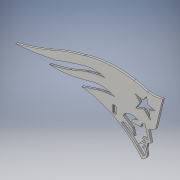
# Autodesk Inventor part: RTS patriots
Saved by Autodesk Inventor 2016 (Build 200138000, 138)
## iProperties
Created: 2017-12-19
Part Number: RTS patriots
Material: Generic
Document SubType Name: Modeling
Designer: student
Density: 1 g/cm^3
Appearance: Default
Author: student
Autodesk Inventor part; units mm, degrees
ref_plane "YZ Plane" through (0, 0, 0) normal (1, 0, 0) x (0, 1, 0)
ref_plane "XZ Plane" through (0, 0, 0) normal (0, 1, 0) x (-1, 0, 0)
ref_plane "XY Plane" through (0, 0, 0) normal (0, 0, 1) x (1, 0, 0)
sketch "Sketch1" plane through (0, 0, 0) normal (0, 0, 1) x (1, 0, 0)
  line L0 (-121.92, 53.34) -> (121.92, 53.34)
  line L1 (121.92, 53.34) -> (121.92, -53.34)
  line L2 (121.92, -53.34) -> (-121.92, -53.34)
  line L3 (-121.92, -53.34) -> (-121.92, 53.34)
  line L4 (-121.92, 53.34) -> (121.92, -53.34) construction
  line L5 (121.92, 53.34) -> (-121.92, -53.34) construction
  arc A0 (67.5496, -52.2242) -> (-16.5252, -5.911) centre (-36.2594, -141.2049) ccw
  arc A1 (67.5496, -52.2242) -> (78.4495, -31.764) centre (64.7451, -37.5966) ccw
  arc A2 (-20.2647, 1.2126) -> (-16.5252, -5.911) centre (-17.1494, -1.6953) ccw
  arc A3 (-43.7287, -2.3938) -> (-20.2647, 1.2126) centre (-53.1153, 136.8126) ccw
  arc A4 (-61.5471, -2.0063) -> (-43.7287, -2.3938) centre (-51.0941, 68.8006) ccw
  arc A5 (-65.9278, 3.1159) -> (-61.5471, -2.0063) centre (-61.6241, 2.3622) ccw
  arc A6 (-108.1597, -0.5066) -> (-65.9278, 3.1159) centre (-96.2599, 108.7489) ccw
  arc A7 (-109.606, 7.2871) -> (-108.1597, -0.5066) centre (-107.7116, 3.6077) ccw
  arc A8 (-109.606, 7.2871) -> (-29.7712, 36.4682) centre (-485.0256, 1158.173) ccw
  arc A9 (46.8022, 47.5707) -> (-29.7712, 36.4682) centre (33.6127, -131.0759) ccw
  arc A10 (75.8647, 41.5807) -> (46.8022, 47.5707) centre (24.6007, -133.6461) ccw
  arc A11 (75.8647, 41.5807) -> (97.0333, 43.8681) centre (82.7984, 76.5092) ccw
  arc A12 (101.3733, 39.6116) -> (97.0333, 43.8681) centre (98.7975, 41.3261) ccw
  line L6 (101.3733, 39.6116) -> (91.2149, -4.1951)
  line L7 (91.2149, -4.1951) -> (82.1219, -9.828)
  line L8 (82.1219, -9.828) -> (85.6883, -23.6524)
  line L9 (85.6883, -23.6524) -> (79.8094, -27.2942)
  line L10 (79.8094, -27.2942) -> (78.4495, -31.764)
  arc A13 (-8.123, 25.7478) -> (-50.7898, 11.8734) centre (130.1222, -471.929) ccw
  arc A14 (-59.7387, 2.1709) -> (-25.343, 4.6976) centre (-51.96, 131.6592) ccw
  arc A15 (-25.343, 4.6976) -> (-3.3955, 10.2777) centre (-241.5674, 901.0891) ccw
  arc A16 (-59.7387, 2.1709) -> (-30.5588, 10.2777) centre (-108.6142, 234.6643) ccw
  arc A17 (-6.8927, 19.9675) -> (-30.5588, 10.2777) centre (128.911, -345.4626) ccw
  arc A18 (29.71, 8.6625) -> (7.2861, 5.2273) centre (28.2796, -56.9055) ccw
  arc A19 (67.5496, -46.6147) -> (-15.043, -2.1204) centre (-26.7986, -122.8453) ccw
  arc A20 (7.2861, 5.2273) -> (-15.043, -2.1204) centre (125.1778, -390.6373) ccw
  arc A21 (29.71, 8.6625) -> (-1.7387, 10.7223) centre (11.2905, -31.4567) ccw
  arc A22 (16.6394, 24.5902) -> (-4.4734, 20.4951) centre (20.0682, -49.5605) ccw
  arc A23 (16.6394, 24.5902) -> (-6.1428, 26.0437) centre (2.4584, -18.4113) ccw
  line L11 (-4.4734, 20.4951) -> (-6.8927, 19.9675)
  line L12 (-1.7387, 10.7223) -> (-3.3955, 10.2777)
  line L13 (-8.123, 25.7478) -> (-6.1428, 26.0437)
  line L14 (-11.9813, 36.4379) -> (-9.4594, 37.5475)
  arc A24 (56.7247, 41.3261) -> (-9.4594, 37.5475) centre (32.0703, -108.3526) ccw
  arc A25 (75.5018, 36.9927) -> (96.2941, 38.7613) centre (82.101, 82.5143) ccw
  arc A26 (75.5018, 36.9927) -> (56.7247, 41.3261) centre (-574.7188, -2737.6346) ccw
  arc A27 (48.5931, -2.1204) -> (42.2239, -8.0879) centre (49.4213, -9.3871) ccw
  arc A28 (62.5792, -3.2945) -> (48.5931, -2.1204) centre (54.4536, -16.199) ccw
  arc A29 (62.5792, -3.2945) -> (53.1895, -9.828) centre (61.8675, -12.2858) ccw
  arc A30 (72.3073, -2.9923) -> (66.2757, -9.3006) centre (72.5246, -9.2377) ccw
  arc A31 (45.1126, -15.108) -> (39.2947, -17.8603) centre (44.2132, -20.7321) ccw
  arc A32 (52.8788, -19.3209) -> (45.1126, -15.108) centre (42.182, -29.7749) ccw
  arc A33 (57.5173, -24.7402) -> (52.8788, -19.3209) centre (-276.2295, -305.7101) ccw
  arc A34 (69.3744, -42.5298) -> (72.1611, -35.7997) centre (66.7227, -37.4899) ccw
  arc A35 (67.5496, -46.6147) -> (73.5131, -32.8714) centre (66.056, -37.8011) ccw
  arc A36 (72.1611, -35.7997) -> (68.1792, -31.764) centre (38.6776, -64.8546) ccw
  arc A37 (69.3744, -42.5298) -> (39.2947, -17.8603) centre (-35.2417, -139.4161) ccw
  line L15 (96.2941, 38.7613) -> (86.6684, -1.6953)
  line L16 (86.6684, -1.6953) -> (76.8032, -7.4567)
  line L17 (76.8032, -7.4567) -> (80.3634, -21.6224)
  line L18 (80.3634, -21.6224) -> (74.9042, -24.8106)
  line L19 (74.9042, -24.8106) -> (74.9042, -28.2436)
  line L20 (74.9042, -28.2436) -> (73.5131, -32.8714)
  line L21 (68.1792, -31.764) -> (71.8142, -31.6183)
  line L22 (71.8142, -31.6183) -> (73.0053, -28.2436)
  line L23 (73.0053, -28.2436) -> (68.1773, -28.4371)
  line L24 (68.1773, -28.4371) -> (63.5764, -30.1012)
  line L25 (63.5764, -30.1012) -> (67.9428, -25.8659)
  line L26 (67.9428, -25.8659) -> (72.4098, -25.6869)
  line L27 (72.4098, -25.6869) -> (72.3107, -23.2165)
  line L28 (72.3107, -23.2165) -> (67.9428, -21.9034)
  line L29 (67.9428, -21.9034) -> (68.8903, -20.251)
  line L30 (68.8903, -20.251) -> (76.5676, -19.9433)
  line L31 (76.5676, -19.9433) -> (72.3073, -2.9923)
  arc A38 (-106.3904, 3.6077) -> (-58.0071, 20.2313) centre (-189.4647, 324.1182) ccw
  arc A39 (-11.9813, 36.4379) -> (-58.0071, 20.2313) centre (40.006, -184.6624) ccw
  line L32 (65.3263, 19.2184) -> (59.2622, 9.8782)
  line L33 (59.2622, 9.8782) -> (70.5776, 13.9377)
  line L34 (70.5776, 13.9377) -> (79.476, 5.0926)
  line L35 (79.476, 5.0926) -> (77.62, 16.6894)
  line L36 (77.62, 16.6894) -> (85.9858, 19.6907)
  line L37 (85.9858, 19.6907) -> (75.851, 22.1929)
  line L38 (75.851, 22.1929) -> (74.2086, 30.8072)
  line L39 (74.2086, 30.8072) -> (68.8903, 24.063)
  line L40 (68.8903, 24.063) -> (58.7931, 26.4044)
  line L41 (58.7931, 26.4044) -> (65.3263, 19.2184)
  line L42 (42.2239, -8.0879) -> (55.0071, -16.3511)
  line L43 (55.0071, -16.3511) -> (57.5173, -24.7402)
  line L44 (53.1895, -9.828) -> (66.2757, -9.3006)
  arc A40 (-106.3904, 3.6077) -> (-50.7898, 11.8734) centre (-136.4008, 396.611) ccw
  line L45 (27.6145, -1.5196) -> (32.0595, -1.5196)
  line L46 (32.0595, -1.5196) -> (32.0595, -11.6796)
  line L47 (32.0595, -11.6796) -> (27.6145, -11.6796)
  line L48 (27.6145, -11.6796) -> (27.6145, -1.5196)
  line L49 (27.6145, -1.5196) -> (32.0595, -11.6796) construction
  line L50 (32.0595, -1.5196) -> (27.6145, -11.6796) construction
  point P0 (0, 0)
  point P1 (29.837, -6.5996)
  dimension "d0" = 243.84
  dimension "d1" = 106.68
  dimension "d21" = 4.445
  dimension "d22" = 10.16
  constraints: 102 end point, 83 point on circle, 41 centre point, 11 parallel, 4 midpoint, 4 perpendicular, 2 horizontal, 1 point on line, 1 tangent, 1 vertical
  measures "d0" distance of L1.end L2.end
  measures "d1" distance of L0.end L1.end
  measures "d21" distance of L46.end L47.end
  measures "d22" distance of L45.end L46.end
extrude "Extrusion2" add sketch "Sketch1" along normal blind 2.54 contours A13 A40 A38 A39 L14 A24 A26 A25 L15 L16 L17 L18 L19 L20 A35 A19 A20 A18 A21 L12 A15 A14 A16 A17 L11 A22 A23 L13
body "Solid2"
